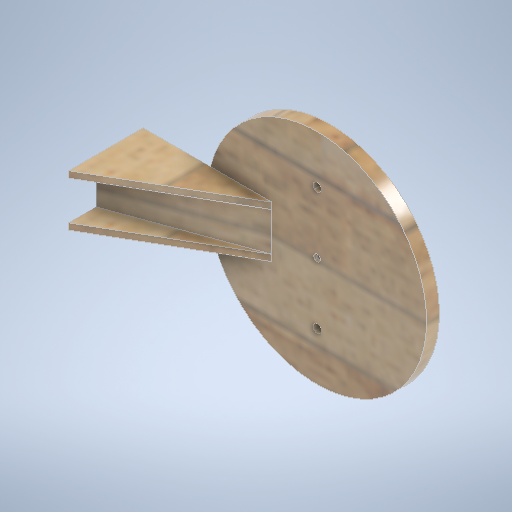
# Autodesk Inventor part: Base
Saved by Autodesk Inventor 2025.3 (Build 293356000, 356)
## iProperties
Created: 2026-03-02
Part Number: Base
Material: Wood (Maple)
Document SubType Name: Modeling
Designer: abdul
Density: 0.67 g/cm^3
Appearance: Natural Maple - Glossy Dark Tint
Author: abdul
Autodesk Inventor part; units mm, degrees
ref_plane "YZ Plane" through (0, 0, 0) normal (1, 0, 0) x (0, 1, 0)
ref_plane "XY Plane" through (0, 0, 0) normal (0, 0, 1) x (1, 0, 0)
sketch "Sketch1" plane through (0, 0, 0) normal (0, 0, 1) x (1, 0, 0)
  circle A0 centre (0, 0) radius 85
  line L0 (0, -85) -> (0, 85)
  line L1 (-85, 0) -> (85, 0)
  circle A1 centre (0, -47.5) radius 3.175
  circle A2 centre (0, 47.5) radius 3.175
  dimension "d0" = 170
  dimension "d21" = 6.35
  dimension "d22" = 47.5
  constraints: 4 end point, 3 centre point, 2 midpoint, 2 point on circle, 1 coincident, 1 horizontal, 1 point on line, 1 symmetric about line, 1 vertical, 1 other
  measures "d0" diameter of A0
  measures "d21" diameter of A1
  measures "d22" vertical distance of L1.end A1.centre
extrude "Extrusion1" add sketch "Sketch1" along normal blind 10
sketch "Sketch2" plane through (0, 0, 0) normal (0, 0, -1) x (-1, 0, 0)
  line L0 (-20, -25) -> (20, -25)
  line L1 (20, -25) -> (20, 25)
  line L2 (20, 25) -> (-20, 25)
  line L3 (-20, 25) -> (-20, -25)
  line L4 (0, -25) -> (0, 25)
  line L5 (5.3, -25) -> (5.3, 25)
  line L6 (-5.3, -25) -> (-5.3, 25)
  circle A0 centre (0, 0) radius 1.5
  point P0 (-5.3, -25)
  point P1 (5.3, -25)
  dimension "d3" = 40
  dimension "d4" = 50
  dimension "d18" = 3
  dimension "d25" = 5.3
  dimension "d27" = 10.6
  constraints: 14 end point, 6 parallel, 3 midpoint, 2 coincident, 2 perpendicular, 2 point on line, 1 centre point, 1 horizontal
  measures "d3" distance of L1.end L2.end
  measures "d4" distance of L0.end L1.end
  measures "d18" diameter of A0
  measures "d25" distance from line of point (0, 0) L5
  measures "d27" distance between parallel lines of L5 L6
extrude "Extrusion2" add sketch "Sketch2" along normal blind 3 contours L3 L2 L6 L0 | L5 L2 L1 L0
extrude "Extrusion3" add sketch "Sketch2" along normal blind 0.5 contours L6 L2 L4 A0 L0 | L4 A0 L2 L5 L0 | A0 L4 | L4 A0
extrude "Extrusion4" cut sketch "Sketch2" along normal through all both and the other way through all contours A0 L4 | L4 A0
extrude "Extrusion5" cut sketch "Sketch1" along normal through all contours A2 L0 | L0 A2 | A1 L0 | L0 A1
thread "Thread1" size "M3x0.5" class "6H" standard "ANSI Metric M Profile" length 77
sketch "Sketch3" plane through (0, 0, 10) normal (0, 0, 1) x (1, 0, 0)
  circle A0 centre (0, 0) radius 2.6
  dimension "d30" = 5.2
  constraints: 1 centre point, 1 coincident
  measures "d30" diameter of A0
extrude "Extrusion6" cut sketch "Sketch3" against normal blind 1.7
ref_plane "Work Plane1" through (0, 15, 0) normal (0, 1, 0) x (-1, 0, 0)
ref_plane "Work Plane2" through (0, -15, 0) normal (0, 1, 0) x (-1, 0, 0)
sketch "Sketch4" plane through (0, 15, 0) normal (0, 1, 0) x (-1, 0, 0)
  line L0 (-20, 0) -> (-83.666, 0) projected
  line L1 (-83.666, 0) -> (-83.666, 10) projected
  line L2 (-83.666, 10) -> (83.666, 10) projected
  line L3 (83.666, 10) -> (83.666, 0) projected
  line L4 (83.666, 0) -> (20, 0) projected
  line L5 (20, 0) -> (20, -3) projected
  line L6 (20, -3) -> (5.3, -3) projected
  line L7 (5.3, -3) -> (5.3, -0.5) projected
  line L8 (5.3, -0.5) -> (-5.3, -0.5) projected
  line L9 (-5.3, -0.5) -> (-5.3, -3) projected
  line L10 (-5.3, -3) -> (-20, -3) projected
  line L11 (-20, -3) -> (-20, 0) projected
  line L12 (85, 10) -> (-85, 10) projected
  line L13 (85, 10) -> (-85, 10) projected
  line L14 (85, 0) -> (-85, 0) projected
  line L15 (35, 10) -> (135, 67.735)
  line L16 (135, 67.735) -> (135, 10)
  line L17 (35, 10) -> (135, 10)
  line L18 (-20, 0) -> (-83.666, 0) projected
  line L19 (-83.666, 0) -> (-83.666, 10) projected
  line L20 (-83.666, 10) -> (83.666, 10) projected
  line L21 (83.666, 10) -> (83.666, 0) projected
  line L22 (83.666, 0) -> (20, 0) projected
  line L23 (20, 0) -> (20, -3) projected
  line L24 (20, -3) -> (5.3, -3) projected
  line L25 (5.3, -3) -> (5.3, -0.5) projected
  line L26 (5.3, -0.5) -> (-5.3, -0.5) projected
  line L27 (-5.3, -0.5) -> (-5.3, -3) projected
  line L28 (-5.3, -3) -> (-20, -3) projected
  line L29 (-20, -3) -> (-20, 0) projected
  point P0 (0, 0)
  dimension "d35" = 30
  dimension "d37" = 100
  dimension "d46" = 35
  constraints: 6 end point, 2 perpendicular, 2 point on line
  measures "d35" angle of L2 L15
  measures "d37" distance of L15.start L16.end
  measures "d46" horizontal distance of point (0, 0) L15.start
extrude "Extrusion7" add sketch "Sketch4" along normal blind 5 contours L15 L16 L17 L12 L2
mirror "Mirror1" about plane through (0, 0, 0) normal (0, 1, 0) of "Extrusion7"
sketch "Sketch5" plane through (0, 0, 0) normal (0, 1, 0) x (-1, 0, 0)
  line L0 (85, 0) -> (20, 0) projected
  line L1 (20, 0) -> (20, -3) projected
  line L2 (20, -3) -> (5.3, -3) projected
  line L3 (5.3, -3) -> (5.3, -0.5) projected
  line L4 (5.3, -0.5) -> (1.5, -0.5) projected
  line L5 (1.5, -0.5) -> (1.5, 8.3) projected
  line L6 (1.5, 8.3) -> (2.6, 8.3) projected
  line L7 (2.6, 8.3) -> (2.6, 10) projected
  line L8 (2.6, 10) -> (85, 10) projected
  line L9 (85, 10) -> (85, 0) projected
  line L10 (-20, 0) -> (-85, 0) projected
  line L11 (-85, 0) -> (-85, 10) projected
  line L12 (-85, 10) -> (-2.6, 10) projected
  line L13 (-2.6, 10) -> (-2.6, 8.3) projected
  line L14 (-2.6, 8.3) -> (-1.5, 8.3) projected
  line L15 (-1.5, 8.3) -> (-1.5, -0.5) projected
  line L16 (-1.5, -0.5) -> (-5.3, -0.5) projected
  line L17 (-5.3, -0.5) -> (-5.3, -3) projected
  line L18 (-5.3, -3) -> (-20, -3) projected
  line L19 (-20, -3) -> (-20, 0) projected
  line L20 (35, 10) -> (135, 46.397)
  line L21 (35, 10) -> (135, 10)
  line L22 (135, 10) -> (135, 46.397)
  line L23 (82.6136, 10) -> (-85, 10) projected
  line L24 (85, 0) -> (20, 0) projected
  line L25 (20, 0) -> (20, -3) projected
  line L26 (20, -3) -> (5.3, -3) projected
  line L27 (5.3, -3) -> (5.3, -0.5) projected
  line L28 (5.3, -0.5) -> (1.5, -0.5) projected
  line L29 (1.5, -0.5) -> (1.5, 8.3) projected
  line L30 (1.5, 8.3) -> (2.6, 8.3) projected
  line L31 (2.6, 8.3) -> (2.6, 10) projected
  line L32 (2.6, 10) -> (85, 10) projected
  line L33 (85, 10) -> (85, 0) projected
  line L34 (-20, 0) -> (-85, 0) projected
  line L35 (-85, 0) -> (-85, 10) projected
  line L36 (-85, 10) -> (-2.6, 10) projected
  line L37 (-2.6, 10) -> (-2.6, 8.3) projected
  line L38 (-2.6, 8.3) -> (-1.5, 8.3) projected
  line L39 (-1.5, 8.3) -> (-1.5, -0.5) projected
  line L40 (-1.5, -0.5) -> (-5.3, -0.5) projected
  line L41 (-5.3, -0.5) -> (-5.3, -3) projected
  line L42 (-5.3, -3) -> (-20, -3) projected
  line L43 (-20, -3) -> (-20, 0) projected
  point P0 (0, 0)
  dimension "d41" = 90
  dimension "d42" = 100
  dimension "d43" = 35
  dimension "d44" = 20
  dimension "d45" = 0
  constraints: 6 end point, 1 parallel
  measures "d41" angle of L22 L21
  measures "d42" distance of L20.start L21.end
  measures "d43" horizontal distance of point (0, 0) L20.start
  measures "d44" angle of L23 L20
  measures "d45" distance from line of L8.end L21
extrude "Extrusion8" add sketch "Sketch5" along normal mid plane 30 contours L8 L20 L22 L21
body "Solid1"
